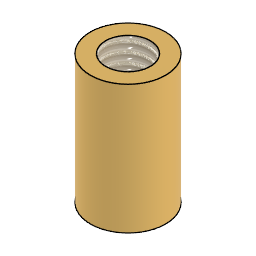
HeatSetInsert-M2.5x6_v1 (Autodesk Fusion 360 design; units mm, degrees)
Autodesk Fusion 360 part; units mm, degrees
sketch "Sketch1" plane through (0, 0, 0) normal (0, 0, 1) x (1, 0, 0)
  circle A0 centre (0, 0) radius 1.75
  circle A1 centre (0, 0) radius 1.25
  dimension "d1" = 3.5
  dimension "d2" = 2.5
  constraint coincident A0.centre A1.centre
  measures "d1" diameter of A0
  measures "d2" diameter of A1
extrude "Extrude1" add sketch "Sketch1" along normal blind 6
thread "Thread1" "ISO Metric profile 2.5 M2.5x0.45 M2.5x0.45 6H" major diameter 2.58 minor diameter 2.0755 pitch 0.45 angle 60 resizes the face on face at (1.2484, -0.0623, 4)
